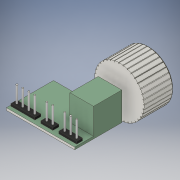
# Autodesk Inventor part: GF1002
Saved by Autodesk Inventor 2018.3 (Build 223284000, 284)
## iProperties
Created: 2018-06-03
Part Number: GF1002
Material: Generisch
Document SubType Name: Modeling
Designer: JochenAlt
Density: 1 g/cm^3
Appearance: Stahl
Author: JochenAlt
Autodesk Inventor part; units mm, degrees
ref_plane "YZ Plane" through (0, 0, 0) normal (1, 0, 0) x (0, 1, 0)
ref_plane "XZ Plane" through (0, 0, 0) normal (0, 1, 0) x (-1, 0, 0)
ref_plane "XY Plane" through (0, 0, 0) normal (0, 0, 1) x (1, 0, 0)
sketch "Skizze1" plane through (0, 0, 0) normal (0, 0, 1) x (1, 0, 0)
  line L0 (-7.1465, 17.3258) -> (21.8535, 17.3258)
  line L1 (21.8535, 17.3258) -> (21.8535, -2.6742)
  line L2 (21.8535, -2.6742) -> (-7.1465, -2.6742)
  line L3 (-7.1465, -2.6742) -> (-7.1465, 17.3258)
  line L4 (-6.7165, 1.3258) -> (3.4435, 1.3258)
  line L5 (3.4435, 1.3258) -> (3.4435, -1.1742)
  line L6 (3.4435, -1.1742) -> (-6.7165, -1.1742)
  line L7 (-6.7165, -1.1742) -> (-6.7165, 1.3258)
  circle A0 centre (-5.4465, 0.0758) radius 0.35
  line L8 (-6.7165, 0.0758) -> (3.4435, 0.0758) construction
  circle A1 centre (-2.9065, 0.0758) radius 0.35
  circle A2 centre (-0.3665, 0.0758) radius 0.35
  circle A3 centre (2.1735, 0.0758) radius 0.35
  line L9 (5.9835, 1.3258) -> (11.0635, 1.3258)
  line L10 (11.0635, 1.3258) -> (11.0635, -1.1742)
  line L11 (11.0635, -1.1742) -> (5.9835, -1.1742)
  line L12 (5.9835, -1.1742) -> (5.9835, 1.3258)
  line L13 (13.6035, 1.3258) -> (21.2235, 1.3258)
  line L14 (21.2235, 1.3258) -> (21.2235, -1.1742)
  line L15 (21.2235, -1.1742) -> (13.6035, -1.1742)
  line L16 (13.6035, -1.1742) -> (13.6035, 1.3258)
  circle A4 centre (7.2535, 0.0758) radius 0.35
  circle A5 centre (14.8735, 0.0758) radius 0.35
  circle A6 centre (9.7935, 0.0758) radius 0.35
  circle A7 centre (17.4135, 0.0758) radius 0.35
  circle A8 centre (19.9535, 0.0758) radius 0.35
  line L17 (21.8535, 17.3258) -> (11.8535, 17.3258)
  line L18 (11.8535, 17.3258) -> (11.8535, 5.3258)
  line L19 (11.8535, 5.3258) -> (21.8535, 5.3258)
  line L20 (21.8535, 5.3258) -> (21.8535, 17.3258)
  point P0 (0, 0)
  dimension "d0" = 29
  dimension "d1" = 20
  dimension "d2" = 0.7
  dimension "d3" = 2.5
  dimension "d5" = 1.27
  dimension "d9" = 2.54
  dimension "d14" = 10.16
  dimension "d16" = 1.5
  dimension "d17" = 1.7
  dimension "d18" = 12.7
  dimension "d21" = 2.54
  dimension "d28" = 2.54
  dimension "d33" = 20.32
  dimension "d34" = 1.27
  dimension "d35" = 1.27
  dimension "d36" = 5.08
  dimension "d37" = 7.62
  dimension "d46" = 10
  dimension "d47" = 12
  constraints: 42 end point, 10 parallel, 9 centre point, 8 horizontal, 5 perpendicular, 2 equal radius, 2 midpoint, 12 other
  measures "d0" distance of L1.end L2.end
  measures "d1" distance of L0.end L1.end
  measures "d2" diameter of A0
  measures "d3" distance of L4.end L5.end
  measures "d5" distance from line of L7 A0.centre
  measures "d9" distance of A0.centre A1.centre
  measures "d14" distance between parallel lines of L5 L7
  measures "d16" distance between parallel lines of L2 L6
  measures "d17" distance from line of L3 A0.centre
  measures "d18" distance of A4.centre A0.centre
  measures "d21" distance of A4.centre A6.centre
  measures "d28" distance of A5.centre A7.centre
  measures "d33" distance of A5.centre A0.centre
  measures "d34" distance from line of L12 A4.centre
  measures "d35" distance from line of L16 A5.centre
  measures "d36" distance of L9.start L9.end
  measures "d37" distance of L13.start L13.end
  measures "d46" distance of L19.end L18.end
  measures "d47" distance of L18.end L17.end
extrude "Extrusion1" add sketch "Skizze1" along normal blind 1 contours L0 L18 L19 L1 L2 L3 | L0 L1 L19 L18 | L4 L5 L6 L7 | L9 L10 L11 L12 | L13 L14 L15 L16
extrude "Extrusion2" add sketch "Skizze1" along normal blind 1 from surface at 1 contours L4 L5 L6 L7 | L9 L10 L11 L12 | L13 L14 L15 L16
extrude "Extrusion3" add sketch "Skizze1" along normal blind 7 and the other way blind 3 from surface at 2 contours A0 | A1 | A2 | A3 | A4 | A5 | A6 | A7 | A8
extrude "Extrusion4" add sketch "Skizze1" along normal blind 12 contours L0 L1 L19 L18
sketch "Skizze2" plane through (-7.1465, 17.3258, 0) normal (0, 1, 0) x (1, 0, 0)
  line L0 (29, -12) -> (19, -12) construction
  line L1 (29, 0) -> (29, -12) construction
  line L2 (19, -1) -> (19, -12) construction
  circle A0 centre (24, -7) radius 1
  circle A1 centre (24, -7) radius 10 construction
  line L3 (23.8018, -16.998) -> (23.6571, -17.498)
  line L4 (23.6571, -17.498) -> (22.1037, -17.331)
  line L5 (22.1037, -17.331) -> (22.0686, -16.8117)
  line L6 (22.8804, -17.4145) -> (24, -7) construction
  line L7 (24, -12) -> (24, -6) construction
  line L8 (23.8018, -16.998) -> (24, -7)
  line L9 (24, -7) -> (22.0686, -16.8117)
  line L10 (25.5409, -16.8806) -> (25.4853, -17.3981)
  line L11 (25.5409, -16.8806) -> (24, -7)
  line L12 (25.4853, -17.3981) -> (23.9265, -17.5034)
  line L13 (23.9265, -17.5034) -> (23.8018, -16.998)
  line L14 (24, -7) -> (23.8018, -16.998)
  line L15 (27.2333, -16.4629) -> (27.2683, -16.9822)
  line L16 (27.2333, -16.4629) -> (24, -7)
  line L17 (27.2683, -16.9822) -> (25.7515, -17.3566)
  line L18 (25.7515, -17.3566) -> (25.5409, -16.8806)
  line L19 (24, -7) -> (25.5409, -16.8806)
  line L20 (28.8273, -15.7577) -> (28.9521, -16.263)
  line L21 (28.8273, -15.7577) -> (24, -7)
  line L22 (28.9521, -16.263) -> (27.5233, -16.8951)
  line L23 (27.5233, -16.8951) -> (27.2333, -16.4629)
  line L24 (24, -7) -> (27.2333, -16.4629)
  line L25 (30.2748, -14.7864) -> (30.4853, -15.2624)
  line L26 (30.2748, -14.7864) -> (24, -7)
  line L27 (30.4853, -15.2624) -> (29.188, -16.1329)
  line L28 (29.188, -16.1329) -> (28.8273, -15.7577)
  line L29 (24, -7) -> (28.8273, -15.7577)
  line L30 (31.5315, -13.5785) -> (31.8216, -14.0107)
  line L31 (31.5315, -13.5785) -> (24, -7)
  line L32 (31.8216, -14.0107) -> (30.6951, -15.0933)
  line L33 (30.6951, -15.0933) -> (30.2748, -14.7864)
  line L34 (24, -7) -> (30.2748, -14.7864)
  line L35 (32.5594, -12.1707) -> (32.9201, -12.546)
  line L36 (32.5594, -12.1707) -> (24, -7)
  line L37 (32.9201, -12.546) -> (31.9988, -13.8077)
  line L38 (31.9988, -13.8077) -> (31.5315, -13.5785)
  line L39 (24, -7) -> (31.5315, -13.5785)
  line L40 (33.3273, -10.6058) -> (33.7477, -10.9127)
  line L41 (33.3273, -10.6058) -> (24, -7)
  line L42 (33.7477, -10.9127) -> (33.0594, -12.3153)
  line L43 (33.0594, -12.3153) -> (32.5594, -12.1707)
  line L44 (24, -7) -> (32.5594, -12.1707)
  line L45 (33.8117, -8.9314) -> (34.279, -9.1606)
  line L46 (33.8117, -8.9314) -> (24, -7)
  line L47 (34.279, -9.1606) -> (33.8448, -10.6614)
  line L48 (33.8448, -10.6614) -> (33.3273, -10.6058)
  line L49 (24, -7) -> (33.3273, -10.6058)
  line L50 (33.998, -7.1982) -> (34.498, -7.3429)
  line L51 (33.998, -7.1982) -> (24, -7)
  line L52 (34.498, -7.3429) -> (34.331, -8.8963)
  line L53 (34.331, -8.8963) -> (33.8117, -8.9314)
  line L54 (24, -7) -> (33.8117, -8.9314)
  line L55 (33.8806, -5.4591) -> (34.3981, -5.5147)
  line L56 (33.8806, -5.4591) -> (24, -7)
  line L57 (34.3981, -5.5147) -> (34.5034, -7.0735)
  line L58 (34.5034, -7.0735) -> (33.998, -7.1982)
  line L59 (24, -7) -> (33.998, -7.1982)
  line L60 (33.4629, -3.7667) -> (33.9822, -3.7317)
  line L61 (33.4629, -3.7667) -> (24, -7)
  line L62 (33.9822, -3.7317) -> (34.3566, -5.2485)
  line L63 (34.3566, -5.2485) -> (33.8806, -5.4591)
  line L64 (24, -7) -> (33.8806, -5.4591)
  line L65 (32.7577, -2.1727) -> (33.263, -2.0479)
  line L66 (32.7577, -2.1727) -> (24, -7)
  line L67 (33.263, -2.0479) -> (33.8951, -3.4767)
  line L68 (33.8951, -3.4767) -> (33.4629, -3.7667)
  line L69 (24, -7) -> (33.4629, -3.7667)
  line L70 (31.7864, -0.7252) -> (32.2624, -0.5147)
  line L71 (31.7864, -0.7252) -> (24, -7)
  line L72 (32.2624, -0.5147) -> (33.1329, -1.812)
  line L73 (33.1329, -1.812) -> (32.7577, -2.1727)
  line L74 (24, -7) -> (32.7577, -2.1727)
  line L75 (30.5785, 0.5315) -> (31.0107, 0.8216)
  line L76 (30.5785, 0.5315) -> (24, -7)
  line L77 (31.0107, 0.8216) -> (32.0933, -0.3049)
  line L78 (32.0933, -0.3049) -> (31.7864, -0.7252)
  line L79 (24, -7) -> (31.7864, -0.7252)
  line L80 (29.1707, 1.5594) -> (29.546, 1.9201)
  line L81 (29.1707, 1.5594) -> (24, -7)
  line L82 (29.546, 1.9201) -> (30.8077, 0.9988)
  line L83 (30.8077, 0.9988) -> (30.5785, 0.5315)
  line L84 (24, -7) -> (30.5785, 0.5315)
  line L85 (27.6058, 2.3273) -> (27.9127, 2.7477)
  line L86 (27.6058, 2.3273) -> (24, -7)
  line L87 (27.9127, 2.7477) -> (29.3153, 2.0594)
  line L88 (29.3153, 2.0594) -> (29.1707, 1.5594)
  line L89 (24, -7) -> (29.1707, 1.5594)
  line L90 (25.9314, 2.8117) -> (26.1606, 3.279)
  line L91 (25.9314, 2.8117) -> (24, -7)
  line L92 (26.1606, 3.279) -> (27.6614, 2.8448)
  line L93 (27.6614, 2.8448) -> (27.6058, 2.3273)
  line L94 (24, -7) -> (27.6058, 2.3273)
  line L95 (24.1982, 2.998) -> (24.3429, 3.498)
  line L96 (24.1982, 2.998) -> (24, -7)
  line L97 (24.3429, 3.498) -> (25.8963, 3.331)
  line L98 (25.8963, 3.331) -> (25.9314, 2.8117)
  line L99 (24, -7) -> (25.9314, 2.8117)
  line L100 (22.4591, 2.8806) -> (22.5147, 3.3981)
  line L101 (22.4591, 2.8806) -> (24, -7)
  line L102 (22.5147, 3.3981) -> (24.0735, 3.5034)
  line L103 (24.0735, 3.5034) -> (24.1982, 2.998)
  line L104 (24, -7) -> (24.1982, 2.998)
  line L105 (20.7667, 2.4629) -> (20.7317, 2.9822)
  line L106 (20.7667, 2.4629) -> (24, -7)
  line L107 (20.7317, 2.9822) -> (22.2485, 3.3566)
  line L108 (22.2485, 3.3566) -> (22.4591, 2.8806)
  line L109 (24, -7) -> (22.4591, 2.8806)
  line L110 (19.1727, 1.7577) -> (19.0479, 2.263)
  line L111 (19.1727, 1.7577) -> (24, -7)
  line L112 (19.0479, 2.263) -> (20.4767, 2.8951)
  line L113 (20.4767, 2.8951) -> (20.7667, 2.4629)
  line L114 (24, -7) -> (20.7667, 2.4629)
  line L115 (17.7252, 0.7864) -> (17.5147, 1.2624)
  line L116 (17.7252, 0.7864) -> (24, -7)
  line L117 (17.5147, 1.2624) -> (18.812, 2.1329)
  line L118 (18.812, 2.1329) -> (19.1727, 1.7577)
  line L119 (24, -7) -> (19.1727, 1.7577)
  line L120 (16.4685, -0.4215) -> (16.1784, 0.0107)
  line L121 (16.4685, -0.4215) -> (24, -7)
  line L122 (16.1784, 0.0107) -> (17.3049, 1.0933)
  line L123 (17.3049, 1.0933) -> (17.7252, 0.7864)
  line L124 (24, -7) -> (17.7252, 0.7864)
  line L125 (15.4406, -1.8293) -> (15.0799, -1.454)
  line L126 (15.4406, -1.8293) -> (24, -7)
  line L127 (15.0799, -1.454) -> (16.0012, -0.1923)
  line L128 (16.0012, -0.1923) -> (16.4685, -0.4215)
  line L129 (24, -7) -> (16.4685, -0.4215)
  line L130 (14.6727, -3.3942) -> (14.2523, -3.0873)
  line L131 (14.6727, -3.3942) -> (24, -7)
  line L132 (14.2523, -3.0873) -> (14.9406, -1.6847)
  line L133 (14.9406, -1.6847) -> (15.4406, -1.8293)
  line L134 (24, -7) -> (15.4406, -1.8293)
  line L135 (14.1883, -5.0686) -> (13.721, -4.8394)
  line L136 (14.1883, -5.0686) -> (24, -7)
  line L137 (13.721, -4.8394) -> (14.1552, -3.3386)
  line L138 (14.1552, -3.3386) -> (14.6727, -3.3942)
  line L139 (24, -7) -> (14.6727, -3.3942)
  line L140 (14.002, -6.8018) -> (13.502, -6.6571)
  line L141 (14.002, -6.8018) -> (24, -7)
  line L142 (13.502, -6.6571) -> (13.669, -5.1037)
  line L143 (13.669, -5.1037) -> (14.1883, -5.0686)
  line L144 (24, -7) -> (14.1883, -5.0686)
  line L145 (14.1194, -8.5409) -> (13.6019, -8.4853)
  line L146 (14.1194, -8.5409) -> (24, -7)
  line L147 (13.6019, -8.4853) -> (13.4966, -6.9265)
  line L148 (13.4966, -6.9265) -> (14.002, -6.8018)
  line L149 (24, -7) -> (14.002, -6.8018)
  line L150 (14.5371, -10.2333) -> (14.0178, -10.2683)
  line L151 (14.5371, -10.2333) -> (24, -7)
  line L152 (14.0178, -10.2683) -> (13.6434, -8.7515)
  line L153 (13.6434, -8.7515) -> (14.1194, -8.5409)
  line L154 (24, -7) -> (14.1194, -8.5409)
  line L155 (15.2423, -11.8273) -> (14.737, -11.9521)
  line L156 (15.2423, -11.8273) -> (24, -7)
  line L157 (14.737, -11.9521) -> (14.1049, -10.5233)
  line L158 (14.1049, -10.5233) -> (14.5371, -10.2333)
  line L159 (24, -7) -> (14.5371, -10.2333)
  line L160 (16.2136, -13.2748) -> (15.7376, -13.4853)
  line L161 (16.2136, -13.2748) -> (24, -7)
  line L162 (15.7376, -13.4853) -> (14.8671, -12.188)
  line L163 (14.8671, -12.188) -> (15.2423, -11.8273)
  line L164 (24, -7) -> (15.2423, -11.8273)
  line L165 (17.4215, -14.5315) -> (16.9893, -14.8216)
  line L166 (17.4215, -14.5315) -> (24, -7)
  line L167 (16.9893, -14.8216) -> (15.9067, -13.6951)
  line L168 (15.9067, -13.6951) -> (16.2136, -13.2748)
  line L169 (24, -7) -> (16.2136, -13.2748)
  line L170 (18.8293, -15.5594) -> (18.454, -15.9201)
  line L171 (18.8293, -15.5594) -> (24, -7)
  line L172 (18.454, -15.9201) -> (17.1923, -14.9988)
  line L173 (17.1923, -14.9988) -> (17.4215, -14.5315)
  line L174 (24, -7) -> (17.4215, -14.5315)
  line L175 (20.3942, -16.3273) -> (20.0873, -16.7477)
  line L176 (20.3942, -16.3273) -> (24, -7)
  line L177 (20.0873, -16.7477) -> (18.6847, -16.0594)
  line L178 (18.6847, -16.0594) -> (18.8293, -15.5594)
  line L179 (24, -7) -> (18.8293, -15.5594)
  line L180 (22.0686, -16.8117) -> (21.8394, -17.279)
  line L181 (22.0686, -16.8117) -> (24, -7)
  line L182 (21.8394, -17.279) -> (20.3386, -16.8448)
  line L183 (20.3386, -16.8448) -> (20.3942, -16.3273)
  line L184 (24, -7) -> (20.3942, -16.3273)
  point P0 (7.1465, 0)
  point P1 (24.7059, -17.4507)
  point P2 (26.5099, -17.1694)
  point P3 (28.2377, -16.579)
  point P4 (29.8367, -15.6977)
  point P5 (31.2583, -14.552)
  point P6 (32.4595, -13.1769)
  point P7 (33.4035, -11.614)
  point P8 (34.0619, -9.911)
  point P9 (34.4145, -8.1196)
  point P10 (34.4507, -6.2941)
  point P11 (34.1694, -4.4901)
  point P12 (33.579, -2.7623)
  point P13 (32.6977, -1.1633)
  point P14 (31.552, 0.2583)
  point P15 (30.1769, 1.4595)
  point P16 (28.614, 2.4035)
  point P17 (26.911, 3.0619)
  point P18 (25.1196, 3.4145)
  point P19 (23.2941, 3.4507)
  point P20 (21.4901, 3.1694)
  point P21 (19.7623, 2.579)
  point P22 (18.1633, 1.6977)
  point P23 (16.7417, 0.552)
  point P24 (15.5405, -0.8231)
  point P25 (14.5965, -2.386)
  point P26 (13.9381, -4.089)
  point P27 (13.5855, -5.8804)
  point P28 (13.5493, -7.7059)
  point P29 (13.8306, -9.5099)
  point P30 (14.421, -11.2377)
  point P31 (15.3023, -12.8367)
  point P32 (16.448, -14.2583)
  point P33 (17.8231, -15.4595)
  point P34 (19.386, -16.4035)
  point P35 (21.089, -17.0619)
  dimension "d50" = 2
  dimension "d51" = 5
  dimension "d52" = 20
  dimension "d55" = 0.5
  dimension "d68" = 10
  dimension "d69" = 100
  dimension "d72" = 360
  constraints: 364 end point, 37 coincident, 37 point on line, 2 midpoint, 2 perpendicular, 2 point on circle, 1 centre point, 1 equal length, 1 vertical alignment, 436 other
  measures "d51" distance from line of L0 point (24, -7)
  measures "d52" diameter of A1
  measures "d55" vertical distance of L3.start L3.end
  measures "d68" angle of L9 L8
  measures "d69" angle of L4 L3
extrude "Extrusion6" add sketch "Skizze2" along normal blind 4 contours A0 L51 L56 | L56 L61 A0 | A0 L46 L51 | L61 L66 A0 | L11 A0 L8 | L8 A0 L9 | L16 A0 L11 | L21 A0 L16 | L26 A0 L21 | L31 A0 L26 | L36 A0 L31 | L41 A0 L36 | L46 A0 L41 | L71 A0 L66 | L76 A0 L71 | L81 A0 L76 | L86 A0 L81 | L91 A0 L86 | L96 A0 L91 | L101 A0 L96 | L106 A0 L101 | L111 A0 L106 | L116 A0 L111 | L121 A0 L116 | L126 A0 L121 | L131 A0 L126 | L136 A0 L131 | L141 A0 L136 | L146 A0 L141 | L151 A0 L146 | L156 A0 L151 | L161 A0 L156 | L166 A0 L161 | L171 A0 L166 | L176 A0 L171 | L9 A0 L176
extrude "Extrusion5" add sketch "Skizze2" along normal blind 12 from surface at 4
sketch "Skizze3" plane through (-7.1465, 17.3258, 0) normal (0, 1, 0) x (1, 0, 0)
  circle A0 centre (24.0155, -6.9837) radius 9.4867
  circle A1 centre (24.0155, -6.9837) radius 8.4867
  circle A2 centre (24.0155, -6.9837) radius 10.4867
  point P0 (7.1465, 0)
  dimension "d83" = 1
  dimension "d84" = 1
  constraints: 3 centre point, 2 coincident
  measures "d83" radial gap between concentric circles of A0 A2
  measures "d84" radial gap between concentric circles of A1 A0
extrude "Extrusion7" add sketch "Skizze3" along normal blind 0.5 from surface at 16
chamfer "Fase2" distance 0.4 angle 45 2 edges at (6.3823, 33.8258, 6.9837) (8.3823, 33.8258, 6.9837)
